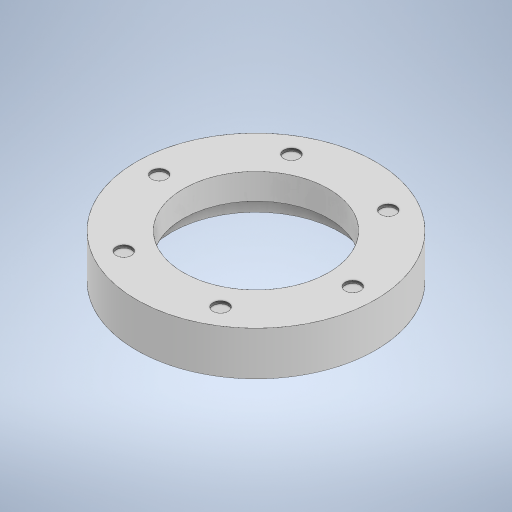
# Autodesk Inventor part: 4_AnilloComplementarioB
Saved by Autodesk Inventor 2024.3 (Build 283343000, 343)
## iProperties
Created: 2024-04-26
Part Number: 4_AnilloComplementarioB
Material: Genérico
Document SubType Name: Modeling
Designer: Cosmic Dinodog
Density: 1 g/cm^3
Appearance: Valor por defecto
Author: Cosmic Dinodog
Autodesk Inventor part; units mm, degrees
ref_plane "YZ Plane" through (0, 0, 0) normal (1, 0, 0) x (0, 1, 0)
ref_plane "XZ Plane" through (0, 0, 0) normal (0, 1, 0) x (-1, 0, 0)
ref_plane "XY Plane" through (0, 0, 0) normal (0, 0, 1) x (1, 0, 0)
sketch "Boceto1" plane through (0, 0, 0) normal (0, 1, 0) x (-1, 0, 0)
  circle A0 centre (0, 0) radius 79
  circle A1 centre (0, 0) radius 48
  dimension "d0" = 158
  dimension "d1" = 96
  constraints: 2 centre point, 2 coincident
  measures "d0" diameter of A0
  measures "d1" diameter of A1
extrude "Extrusión1" add sketch "Boceto1" against normal blind 29
sketch "Boceto2" plane through (0, -29, 0) normal (0, -1, 0) x (1, 0, 0)
  circle A0 centre (0, 0) radius 56
  dimension "d4" = 112
  constraints: 1 centre point, 1 coincident
  measures "d4" diameter of A0
extrude "Extrusión2" cut sketch "Boceto2" against normal blind 12
sketch "Boceto3" plane through (0, 0, 0) normal (0, 1, 0) x (1, 0, 0)
  circle A0 centre (0, 0) radius 64 construction
  circle A1 centre (0, 0) radius 48 projected
  line L0 (0, 0) -> (64, 0) construction
  point P0 (32, 55.4256)
  point P1 (-32, 55.4256)
  point P2 (-64, 0)
  point P3 (-32, -55.4256)
  point P4 (32, -55.4256)
  dimension "d7" = 128
  dimension "d10" = 360
  constraints: 2 coincident, 2 end point, 1 horizontal, 1 horizontal alignment, 9 other
hole "Agujero1" at (64, 0, 0) at (32, 0, -55.4256) at (-32, 0, -55.4256) at (-64, 0, 0) at (-32, 0, 55.4256) at (32, 0, 55.4256) direction (0, -1, 0) diameter 10.106 depth 1.75 thread size "M12x1.75" class "6H" standard "ISO Metric profile"
